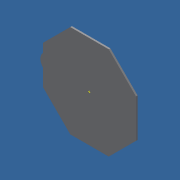
# Autodesk Inventor part: Oktagon_Deckel
Saved by Autodesk Inventor 2018.2 (Build 222227000, 227)
## iProperties
Created: 2018-10-01
Part Number: Oktagon_Deckel
Material: geeigneten Werkstoff auswählen !
Document SubType Name: Modeling
Designer: N.Grubert
Density: 0.001 g/cm^3
Appearance: Vorgabe
Fläche: 0 cm²
Gewicht: 0 g
Dateiname: P:\INVENTOR\Inventor 2018\Templates\ILT\Norm.ipt
Bez_eng: bolt
Bez_french: boulon
Author: N.Grubert
Autodesk Inventor part; units mm, degrees
ref_plane "YZ Plane" through (0, 0, 0) normal (1, 0, 0) x (0, 1, 0)
ref_plane "XZ Plane" through (0, 0, 0) normal (0, 1, 0) x (-1, 0, 0)
ref_plane "XY Plane" through (0, 0, 0) normal (0, 0, 1) x (1, 0, 0)
sketch "Skizze4" plane through (0, 0, 0) normal (0, 1, 0) x (-1, 0, 0)
  line L0 (28.9949, 70) -> (70, 28.9949)
  line L1 (70, 28.9949) -> (70, -28.9949)
  line L2 (70, -28.9949) -> (28.9949, -70)
  line L3 (28.9949, -70) -> (-28.9949, -70)
  line L4 (-28.9949, -70) -> (-70, -28.9949)
  line L5 (-70, -28.9949) -> (-70, 28.9949)
  line L6 (-70, 28.9949) -> (-28.9949, 70)
  line L7 (-28.9949, 70) -> (28.9949, 70)
  line L8 (0, -98) -> (0, 98) construction
  line L9 (98, 0) -> (-98, 0) construction
  point P0 (0, 0)
  point P1 (0, 0)
  dimension "d4" = 140
  constraints: 16 end point, 1 coincident, 18 other
  measures "d4" distance between parallel lines of L3 L7
extrude "Extrusion2" add sketch "Skizze4" along normal blind 2.5
sketch "Skizze9" plane through (0, 2.5, 0) normal (0, 1, 0) x (1, 0, 0)
  line L0 (-70, -28.9949) -> (-28.9949, -70) construction
  line L1 (-28.9949, -70) -> (28.9949, -70) construction
  line L2 (28.9949, -70) -> (70, -28.9949) construction
  line L3 (70, -28.9949) -> (70, 28.9949) construction
  line L4 (70, 28.9949) -> (28.9949, 70) construction
  line L5 (28.9949, 70) -> (-28.9949, 70) construction
  line L6 (-28.9949, 70) -> (-70, 28.9949) construction
  line L7 (-70, 28.9949) -> (-70, -28.9949) construction
  line L8 (-27.7523, -67) -> (-67, -27.7523)
  line L9 (-67, -27.7523) -> (-67, 27.7523)
  line L10 (-67, 27.7523) -> (-27.7523, 67)
  line L11 (-27.7523, 67) -> (27.7523, 67)
  line L12 (27.7523, 67) -> (67, 27.7523)
  line L13 (67, 27.7523) -> (67, -27.7523)
  line L14 (67, -27.7523) -> (27.7523, -67)
  line L15 (27.7523, -67) -> (-27.7523, -67)
  line L16 (-64, -26.5097) -> (-26.5097, -64)
  line L17 (-26.5097, -64) -> (26.5097, -64)
  line L18 (26.5097, -64) -> (64, -26.5097)
  line L19 (64, -26.5097) -> (64, 26.5097)
  line L20 (64, 26.5097) -> (26.5097, 64)
  line L21 (26.5097, 64) -> (-26.5097, 64)
  line L22 (-26.5097, 64) -> (-64, 26.5097)
  line L23 (-64, 26.5097) -> (-64, -26.5097)
  point P0 (0, 0)
  dimension "d20" = 3
  dimension "d21" = 3
  constraints: 32 end point, 14 other
  measures "d20" distance between parallel lines of L0 L8
  measures "d21" distance between parallel lines of L8 L16
extrude "Extrusion6" add sketch "Skizze9" along normal blind 3
sketch "Skizze7" plane through (0, 0, 0) normal (0, -1, 0) x (1, 0, 0)
  line L0 (-28.9949, 70) -> (-70, 28.9949) construction
  line L1 (-70, 28.9949) -> (-70, -28.9949) construction
  line L2 (-70, -28.9949) -> (-28.9949, -70) construction
  line L3 (-28.9949, -70) -> (28.9949, -70) construction
  line L4 (28.9949, -70) -> (70, -28.9949) construction
  line L5 (70, -28.9949) -> (70, 28.9949) construction
  line L6 (70, 28.9949) -> (28.9949, 70) construction
  line L7 (28.9949, 70) -> (-28.9949, 70) construction
  line L8 (-70, 28.9949) -> (-70, -28.9949) projected
  arc A0 (-70, 9.798) -> (-70, -9.798) centre (-60, 0) ccw
  line L9 (-87.767, 0) -> (-49.4975, 0) construction
  line L10 (-78.3477, 9.798) -> (-61.6523, 9.798) construction
  line L11 (-77.7764, -9.798) -> (-65.8218, -9.798) construction
  line L12 (-119.3204, 0) -> (101.5534, 0) construction
  point P0 (0, 0)
  dimension "d15" = 14
  dimension "d16" = 10
  constraints: 6 end point, 4 point on line, 3 horizontal, 3 point on circle, 1 centre point, 1 collinear, 1 midpoint, 1 other
  measures "d15" radius of A0
  measures "d16" distance from line of L1 A0.centre
extrude "Extrusion5" add sketch "Skizze7" against normal up to surface (2.5 mm away)
